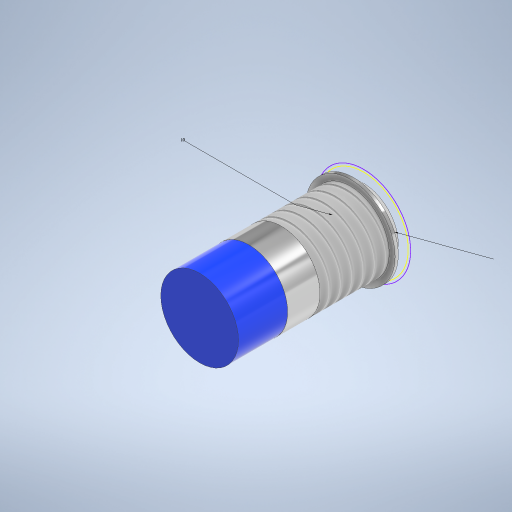
# Autodesk Inventor part: Кнопка
Saved by Autodesk Inventor 2023 (Build 270158000, 158)
## iProperties
Created: 2022-06-07
Part Number: Кнопка
Material: Типовые
Document SubType Name: Modeling
Designer: Admin
Density: 1 g/cm^3
Appearance: По умолчанию
Author: Admin
Autodesk Inventor part; units mm, degrees
ref_plane "YZ Plane" through (0, 0, 0) normal (1, 0, 0) x (0, 1, 0)
ref_plane "XZ Plane" through (0, 0, 0) normal (0, 1, 0) x (-1, 0, 0)
ref_plane "XY Plane" through (0, 0, 0) normal (0, 0, 1) x (1, 0, 0)
sketch "Эскиз1" plane through (0, 0, 0) normal (0, 0, 1) x (1, 0, 0)
  circle A0 centre (0, 0) radius 6.9
  circle A1 centre (0, 0) radius 6
  dimension "d0" = 13.8
  dimension "d2" = 12
  constraints: 3 coincident, 2 centre point
  measures "d0" diameter of A0
  measures "d2" diameter of A1
extrude "Выдавливание1" add sketch "Эскиз1" against normal blind 2 contours A0 | A1
extrude "Выдавливание2" add sketch "Эскиз1" along normal blind 10.7 contours A1
sketch "Эскиз2" plane through (0, 0, 10.7) normal (0, 0, 1) x (1, 0, 0)
  circle A0 centre (0, 0) radius 6 projected
extrude "Выдавливание3" add sketch "Эскиз2" along normal blind 5 separate body
thread "Резьба1" size "M12x1.75" class "6g" standard "ISO Metric profile" length 150
sketch "Эскиз3" plane through (0, 0, 15.7) normal (0, 0, 1) x (1, 0, 0)
  circle A0 centre (0, 0) radius 6 projected
extrude "Выдавливание4" add sketch "Эскиз3" along normal blind 7.6 bodies 1
chamfer "Фаска1" distance 1.5 angle 45 1 edges at (-6.9, 0, -2)
sketch "Эскиз4" plane through (0, 0, -2) normal (0, 0, -1) x (-1, 0, 0)
  circle A0 centre (0, 0) radius 6.9 projected
  circle A1 centre (0, 0) radius 5
  circle A2 centre (0, 0) radius 7.2725
  dimension "d16" = 10
  constraints: 2 centre point, 2 coincident
  measures "d16" diameter of A1
